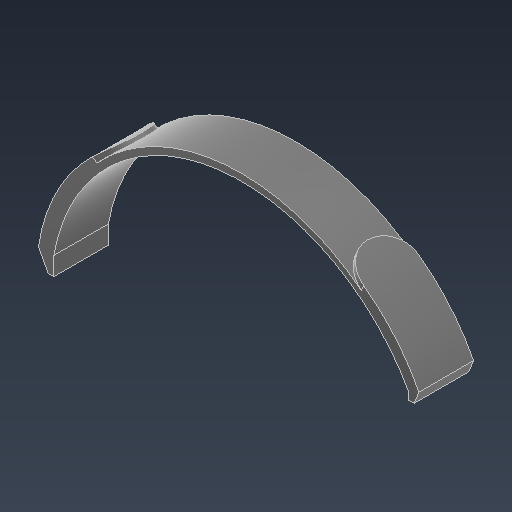
# Autodesk Inventor part: thigh_strap_01
Saved by Autodesk Inventor 2025.2 (Build 292293000, 293)
## iProperties
Created: 2025-03-07
Part Number: thigh_strap_01
Material: Acetal Resin, Black
Document SubType Name: Modeling
Designer: email
Density: 1.425 g/cm^3
Appearance: Smooth - Black
Author: email
Autodesk Inventor part; units mm, degrees
ref_plane "YZ Plane" through (0, 0, 0) normal (1, 0, 0) x (0, 1, 0)
ref_plane "XZ Plane" through (0, 0, 0) normal (0, 1, 0) x (-1, 0, 0)
ref_plane "Work Plane1" through (0, 0, -70) normal (0, 0, 1) x (1, 0, 0)
sketch "Sketch1" plane through (0, 0, -70) normal (0, 0, 1) x (1, 0, 0)
  line L0 (105.135585, -0.094334) -> (105.135585, -23.278359)
  line L1 (-62.514415, -50.241251) -> (-62.514415, -27.759659)
  line L2 (-62.514415, -26.419466) -> (-62.514415, -51.782245)
  line L3 (102.485585, -0.094334) -> (102.485585, -23.278359)
  line L4 (102.485585, 1.408956) -> (105.135585, 1.408956)
  line L5 (-62.514415, -26.419466) -> (-62.514415, -51.782245)
  line L6 (-65.164415, -50.241251) -> (-65.164415, -27.759659)
  line L7 (-62.514415, -26.419466) -> (-65.164415, -26.419466)
  arc A0 (105.135585, 1.408956) -> (-65.164415, -26.419466) centre (24.560741, -40.503573) ccw
  line L8 (-65.164415, -26.419466) -> (-67.161965, -26.419466)
  arc A1 (102.485585, 1.408956) -> (-62.514415, -26.419466) centre (24.895442, -41.61673) ccw
  line L9 (-65.164415, -26.419466) -> (-69.658457, -26.419466)
  arc A2 (-34.319919, 30.819568) -> (-69.658457, -26.419466) centre (14.828678, -39.052317) ccw
  line L10 (-34.319919, 30.819568) -> (-32.803901, 29.911365)
  line L11 (105.135585, 1.408956) -> (107.351745, 3.413316)
  arc A3 (107.351745, 3.413316) -> (70.831931, 40.201852) centre (31.896127, -34.970341) ccw
  line L12 (70.831931, 40.201852) -> (69.891547, 38.198928)
  line L13 (102.485585, 1.408956) -> (102.485585, -2.185128)
  line L14 (102.485585, -2.185128) -> (105.135585, -2.185128)
  line L15 (107.351745, 3.413316) -> (105.135585, -2.185128)
  line L16 (-69.658457, -26.419466) -> (-65.164415, -34.970341)
  line L17 (-65.164415, -34.970341) -> (-62.514415, -34.970341)
  line L18 (-62.514415, -34.970341) -> (-62.514415, -26.419466)
  point P0 (0, 0)
  point P1 (-31.670702, 30.819568)
  constraints: 22 end point, 11 point on circle, 4 centre point, 4 point on line, 3 horizontal, 1 collinear, 1 perpendicular
extrude "Extrusion1" add sketch "Sketch1" along normal blind 25.4
fillet "Fillet1" radius 12.7 4 edges at (-33.5619, 30.3655, -70) (-33.5619, 30.3655, -44.6) (70.3617, 39.2004, -70) (70.3617, 39.2004, -44.6)
body "Solid1"
